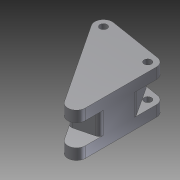
# Autodesk Inventor part: GHI
Saved by Autodesk Inventor 2011 SP2 (Build 150309200, 309)
## iProperties
Created: 2014-05-09
Part Number: GHI
Document SubType Name: Modeling
Designer: Maurice Woods
Density: 1 g/cm^3
Author: Maurice Woods
Autodesk Inventor part; units mm, degrees
ref_plane "YZ Plane" through (0, 0, 0) normal (1, 0, 0) x (0, 1, 0)
ref_plane "XZ Plane" through (0, 0, 0) normal (0, 1, 0) x (-1, 0, 0)
ref_plane "XY Plane" through (0, 0, 0) normal (0, 0, 1) x (1, 0, 0)
sketch "Sketch1" plane through (0, 0, 0) normal (0, 0, 1) x (1, 0, 0)
  line L0 (0, 0) -> (-24.2225, 3.8783) construction
  line L1 (-24.2225, 3.8783) -> (0, -32.7525) construction
  line L2 (0, -32.7525) -> (0, 0) construction
  line L3 (0.6324, 3.9497) -> (-23.5901, 7.828)
  line L4 (-27.559, 1.672) -> (-3.3365, -34.9588)
  line L5 (4, -32.7525) -> (4, 0)
  arc A0 (-23.5901, 7.828) -> (-27.559, 1.672) centre (-24.2225, 3.8783) ccw
  arc A1 (4, 0) -> (0.6324, 3.9497) centre (0, 0) ccw
  arc A2 (-3.3365, -34.9588) -> (4, -32.7525) centre (0, -32.7525) ccw
  dimension "d0" = 32.7525
  dimension "d6" = 24.531
  dimension "d14" = 43.9153
  dimension "d15" = 4
  constraints: 12 end point, 6 point on circle, 6 tangent, 3 centre point, 2 coincident, 2 equal radius, 1 vertical, 2 other
  measures "d0" distance of L1.end L0.start
  measures "d6" distance of L0.start L0.end
  measures "d14" distance of L0.end L1.end
  measures "d15" radius of A0
extrude "Extrusion1" add sketch "Sketch1" along normal mid plane 20
sketch "Sketch2" plane through (0, 0, 0) normal (0, 0, 1) x (1, 0, 0)
  arc A0 (-23.5901, 7.828) -> (-27.559, 1.672) centre (-24.2225, 3.8783) ccw construction
  line L0 (-3.3365, -34.9588) -> (-27.559, 1.672) construction
  arc A1 (-3.3365, -34.9588) -> (4, -32.7525) centre (0, -32.7525) ccw construction
  line L1 (4, 0) -> (4, -32.7525) construction
  arc A2 (4, 0) -> (0.6324, 3.9497) centre (0, 0) ccw construction
  line L2 (-23.5901, 7.828) -> (0.6324, 3.9497) construction
  arc A3 (4, 0) -> (0.6324, 3.9497) centre (0, 0) ccw
  line L3 (4, 0) -> (4, -9.4664)
  arc A4 (-3.3365, -34.9588) -> (4, -32.7525) centre (0, -32.7525) ccw
  line L4 (-3.3365, -34.9588) -> (-7.3441, -28.8984)
  arc A5 (-23.5901, 7.828) -> (-27.559, 1.672) centre (-24.2225, 3.8783) ccw
  line L5 (-23.5901, 7.828) -> (-14.753, 6.4131)
  line L6 (-23.6943, -4.1725) -> (-14.753, 6.4131)
  line L7 (-5.4064, 4.9166) -> (4, -9.4664)
  line L8 (-7.3441, -28.8984) -> (4, -26.0222)
  line L9 (-23.6943, -4.1725) -> (-27.559, 1.672)
  line L10 (-7.3441, -28.8984) -> (-23.6943, -4.1725) construction
  line L11 (4, -9.4664) -> (4, -26.0222) construction
  line L12 (4, -26.0222) -> (4, -32.7525)
  line L13 (-5.4064, 4.9166) -> (0.6324, 3.9497)
  line L14 (-14.753, 6.4131) -> (-5.4064, 4.9166) construction
  constraints: 24 end point, 8 collinear, 6 point on circle, 3 centre point, 3 concentric, 1 point on line
extrude "Extrusion2" cut sketch "Sketch2" along normal mid plane 10
fillet "Fillet1" radius 2 6 edges at (4, -9.4664, 0) (-5.4064, 4.9166, 0) (4, -26.0222, 0) (-7.3441, -28.8984, 0) (-23.6943, -4.1725, 0) (-14.753, 6.4131, 0)
sketch "Sketch3" plane through (0, 0, 10) normal (0, 0, 1) x (1, 0, 0)
  arc A0 (-23.5901, 7.828) -> (-27.559, 1.672) centre (-24.2225, 3.8783) ccw construction
  arc A1 (-3.3365, -34.9588) -> (4, -32.7525) centre (0, -32.7525) ccw construction
  arc A2 (4, 0) -> (0.6324, 3.9497) centre (0, 0) ccw construction
hole "Hole1" at (-24.2225, 3.8783, 10) at (0, 0, 10) direction (0, 0, -1) diameter 3.4 end through all clearance for "Socket Head Cap Screw" size "M3" standard "Ansi Metric M Profile"
equation "\"d0\" = LengthI"
equation "\"d6\" = LengthG"
equation "\"d14\" = LengthH"
equation "\"LengthI\" = 32.752538"
equation "\"LengthG\" = 24.531041"
equation "\"LengthH\" = 43.915254"
body "Solid1"
